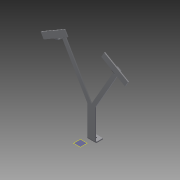
# Autodesk Inventor part: Feeder-Grabber_v2
Saved by Autodesk Inventor 2013 (Build 170138000, 138)
## iProperties
Created: 2013-01-21
Part Number: Feeder-Grabber_v2
Material: Generic
Document SubType Name: Sheet Metal
Designer: motoennies
Density: 1 g/cm^3
Sheet Metal Rule: Default
Author: motoennies
Autodesk Inventor part; units mm, degrees
ref_plane "YZ Plane" through (0, 0, 0) normal (1, 0, 0) x (0, 1, 0)
ref_plane "XZ Plane" through (0, 0, 0) normal (0, 1, 0) x (-1, 0, 0)
ref_plane "XY Plane" through (0, 0, 0) normal (0, 0, 1) x (1, 0, 0)
sketch "Sketch13" plane through (0, 0, 0) normal (0, 0, 1) x (1, 0, 0)
  line L0 (0, 0) -> (25.4, 0)
  line L1 (25.4, 0) -> (25.4, 101.6)
  line L2 (0, 0) -> (0, 101.6)
  line L3 (0, 101.6) -> (-84.322, 247.65)
  line L4 (25.4, 101.6) -> (166.7245, 101.6) construction
  line L5 (25.4, 101.6) -> (109.722, 247.65)
  line L6 (25.4, 101.6) -> (194.044, 101.6) construction
  line L7 (-84.322, 247.65) -> (-73.3235, 254)
  line L8 (109.722, 247.65) -> (98.7235, 254)
  line L9 (-73.3235, 254) -> (12.7, 105.003)
  line L10 (98.7235, 254) -> (12.7, 105.003)
  dimension "d54" = 25.4
  dimension "d55" = 101.6
  dimension "d133" = 60
  dimension "d134" = 150
  dimension "d135" = 12.7
  dimension "d137" = 12.7
  dimension "d139" = 0
  dimension "d140" = 152.4
  dimension "d141" = 152.4
  measures "d54" distance of L0.start L0.end
  measures "d55" distance of L0.end L1.end
  measures "d133" angle of L4 L5
  measures "d134" angle of L2 L3
  measures "d135" distance of L3.end L7.end
  measures "d137" distance of L5.end L8.end
  measures "d139" vertical distance of L1.end L2.end
  measures "d140" vertical distance of L1.end L8.end
  measures "d141" vertical distance of L2.end L7.end
extrude "Plate5" add sketch "Sketch13" along normal blind 3.048
ref_plane "Work Plane1" through (0, 0, 25.4) normal (0, -1, 0) x (1, 0, 0)
sketch "Sketch20" plane through (0, 3.048, 3.048) normal (0, -1, 0) x (1, 0, 0)
  line L0 (25.4, 0) -> (0, 0)
  line L1 (0, 0) -> (0, -25.4)
  line L2 (0, -25.4) -> (25.4, -25.4)
  line L3 (25.4, -25.4) -> (25.4, 0)
  constraints: 6 end point, 1 horizontal, 1 perpendicular, 1 vertical
edge flange "Flange7" height 25.4 angle 90 thickness 3.048 bend radius 3.048 thickness toward (0, -1, 0) relief straight relief width 3.048 relief depth 1.524 edges at (12.7, 0, 0) wall of the first edge with corners at (25.4, 3.048, 3.048) (0, 3.048, 3.048) (0, 3.048, -22.352) (25.4, 3.048, -22.352)
bend "Bend7"
corner "Corner7"
sketch "Sketch21" plane through (0, 0, -22.352) normal (0, -1, 0) x (1, 0, 0)
  line L0 (25.4, 0) -> (0, 0) projected
  line L1 (25.4, 19.304) -> (25.4, 0) projected
  circle A0 centre (12.7, 9.652) radius 2.54
  point P0 (0, 22.352)
  dimension "d123" = 5.08
  dimension "d124" = 12.7
  dimension "d125" = 9.652
  constraints: 1 centre point
  measures "d123" diameter of A0
  measures "d124" distance from line of L1 A0.centre
  measures "d125" distance from line of L0 A0.centre
extrude "Cut3" cut sketch "Sketch21" against normal blind 3.048
sketch "Sketch24" plane through (-82.798, 245.0104, 0) normal (-0.5, 0.8660254, 0) x (-0.8660254, -0.5, 0)
  line L0 (-12.7, 0) -> (0, 0)
  line L1 (0, 0) -> (0, 25.4)
  line L2 (0, 25.4) -> (-12.7, 25.4)
  line L3 (-12.7, 25.4) -> (-12.7, 0)
  constraints: 6 end point, 1 horizontal, 1 perpendicular, 1 vertical
edge flange "Flange8" height 25.4 angle 90 thickness 3.048 bend radius 3.048 thickness toward (-0.5, 0.8660254, 0) relief straight relief width 3.048 relief depth 1.524 corner gap 3.048 corner form 0 edges at (-78.8227, 250.825, 3.048) (104.2227, 250.825, 3.048) wall of the first edge with corners at (-71.7995, 251.3604, 0) (-82.798, 245.0104, 0) (-82.798, 245.0104, 25.4) (-71.7995, 251.3604, 25.4)
bend "Bend8"
corner "Corner8"
sketch "Sketch25" plane through (-71.7995, 251.3604, 22.352) normal (0, 0, 1) x (1, 0, 0)
  line L0 (-10.9985, -6.35) -> (0, 0)
  line L1 (0, 0) -> (-12.7, 21.997)
  line L2 (-12.7, 21.997) -> (-23.6985, 15.647)
  line L3 (-23.6985, 15.647) -> (-10.9985, -6.35)
  constraints: 6 end point, 1 perpendicular, 2 other
edge flange "Flange9" height 25.4 angle 90 thickness 3.048 bend radius 3.048 thickness toward (0, 0, 1) relief straight relief width 3.048 relief depth 1.524 corner gap 3.048 corner form 0 edges at (-78.8227, 250.825, 25.4) (104.2227, 250.825, 25.4) wall of the first edge with corners at (-82.798, 245.0104, 22.352) (-71.7995, 251.3604, 22.352) (-84.4995, 273.3574, 22.352) (-95.498, 267.0074, 22.352)
bend "Bend9"
corner "Corner9"
sketch "Sketch26" plane through (-84.4995, 273.3574, 25.4) normal (0.8660254, 0.5, 0) x (0, 0, -1)
  line L0 (0, -19.304) -> (3.048, -19.304) projected
  line L1 (3.048, 0) -> (3.048, -19.304) projected
  line L2 (3.048, 0) -> (0, 0) projected
  line L3 (0, 0) -> (0, -19.304) projected
  point P0 (25.4, -278.9842)
extrude "Extrusion10" add sketch "Sketch26" along normal blind 38.1
sketch "Sketch27" plane through (120.898, 267.0074, 25.4) normal (0.8660254, -0.5, 0) x (0, 0, -1)
  line L0 (0, -19.304) -> (3.048, -19.304) projected
  line L1 (3.048, 0) -> (3.048, -19.304) projected
  line L2 (3.048, 0) -> (0, 0) projected
  line L3 (0, 0) -> (0, -19.304) projected
  point P0 (25.4, -291.6842)
extrude "Extrusion11" add sketch "Sketch27" along normal blind 38.1
sketch "Sketch28" plane through (-95.498, 267.0074, 22.352) normal (-0.8660254, -0.5, 0) x (0, 0, 1)
  line L0 (0, -19.304) -> (3.048, -19.304) projected
  line L1 (3.048, -19.304) -> (3.048, 0) projected
  line L2 (0, 0) -> (3.048, 0) projected
  line L3 (0, 0) -> (0, -19.304) projected
  point P0 (-22.352, -278.9842)
extrude "Extrusion12" add sketch "Sketch28" along normal blind 38.1
sketch "Sketch29" plane through (109.8995, 273.3574, 22.352) normal (-0.8660254, 0.5, 0) x (0, 0, 1)
  line L0 (0, -19.304) -> (3.048, -19.304) projected
  line L1 (3.048, -19.304) -> (3.048, 0) projected
  line L2 (0, 0) -> (3.048, 0) projected
  line L3 (0, 0) -> (0, -19.304) projected
  point P0 (-22.352, -291.6842)
extrude "Extrusion13" add sketch "Sketch29" along normal blind 38.1
equation "\"d126\" = Thickness"
equation "\"d113\" = BendReliefWidth"
equation "\"d114\" = BendReliefDepth"
equation "\"d115\" = MinimumRemnant"
equation "\"d116\" = BendRadius"
equation "\"d119\" = BendRadius"
equation "\"d120\" = CornerReliefSize"
equation "\"d121\" = GapSize"
equation "\"d122\" = JacobiRadiusSize"
equation "\"d142\" = BendReliefWidth"
equation "\"d143\" = BendReliefDepth"
equation "\"d144\" = MinimumRemnant"
equation "\"d145\" = BendRadius"
equation "\"d148\" = BendRadius"
equation "\"d149\" = CornerReliefSize"
equation "\"d150\" = GapSize"
equation "\"d151\" = JacobiRadiusSize"
equation "\"d152\" = BendReliefWidth"
equation "\"d153\" = BendReliefDepth"
equation "\"d154\" = MinimumRemnant"
equation "\"d155\" = BendRadius"
equation "\"d158\" = BendRadius"
equation "\"d159\" = CornerReliefSize"
equation "\"d160\" = GapSize"
equation "\"d161\" = JacobiRadiusSize"
equation "\"BendRadius\" = Thickness"
equation "\"BendReliefWidth\" = Thickness"
equation "\"BendReliefDepth\" = 0.5 * Thickness"
equation "\"CornerReliefSize\" = 4 * Thickness"
equation "\"MinimumRemnant\" = 2 * Thickness"
equation "\"TransitionRadius\" = BendRadius"
equation "\"JacobiRadiusSize\" = BendRadius"
equation "\"GapSize\" = Thickness"
equation "\"d2\" = BendRadius"
equation "\"d69\" = BendRadius"
equation "\"Thickness\" = 3.048"
body "Solid3"
